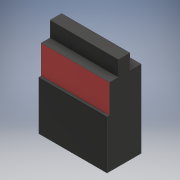
# Autodesk Inventor part: Battery_278Wh
Saved by Autodesk Inventor 2017 (Build 210142000, 142)
## iProperties
Created: 2019-06-03
Part Number: Battery_278Wh
Material: ABS Plastic
Document SubType Name: Modeling
Designer: Dell
Density: 1.06 g/cm^3
Appearance: Smooth - Black
Author: Dell
Autodesk Inventor part; units mm, degrees
ref_plane "YZ Plane" through (0, 0, 0) normal (1, 0, 0) x (0, 1, 0)
ref_plane "XZ Plane" through (0, 0, 0) normal (0, 1, 0) x (-1, 0, 0)
ref_plane "XY Plane" through (0, 0, 0) normal (0, 0, 1) x (1, 0, 0)
sketch "Sketch1" plane through (0, 0, 0) normal (0, 0, 1) x (1, 0, 0)
  line L0 (0, 0) -> (177.8, 0)
  line L1 (177.8, 0) -> (177.8, 88.9)
  line L2 (177.8, 88.9) -> (0, 88.9)
  line L3 (0, 88.9) -> (0, 0)
  dimension "d0" = 88.9
  dimension "d1" = 177.8
  constraints: 8 end point, 2 parallel, 1 horizontal, 1 perpendicular
  measures "d0" distance of L2.end L0.start
  measures "d1" distance of L1.end L2.end
extrude "Extrusion1" add sketch "Sketch1" along normal blind 241.3
sketch "Sketch2" plane through (0, 0, 0) normal (0, -1, 0) x (1, 0, 0)
  line L0 (0, 0) -> (0, 241.3) projected
  line L1 (177.8, 0) -> (177.8, 241.3) projected
  line L2 (0, 203.2) -> (177.8, 203.2)
  line L3 (177.8, 203.2) -> (177.8, 127)
  line L4 (177.8, 127) -> (0, 127)
  line L5 (0, 127) -> (0, 203.2)
  line L6 (0, 0) -> (177.8, 0) projected
  dimension "d4" = 203.2
  dimension "d5" = 127
  constraints: 8 end point, 2 parallel, 2 point on line, 1 horizontal, 1 perpendicular
  measures "d4" distance between parallel lines of L6 L2
  measures "d5" distance between parallel lines of L6 L4
extrude "Extrusion2" cut sketch "Sketch2" against normal blind 6.35 contours L0 L2 L1 L4
sketch "Sketch3" plane through (0, 0, 241.3) normal (0, 0, 1) x (1, 0, 0)
  line L0 (177.8, 0) -> (177.8, 88.9) projected
  line L1 (0, 0) -> (177.8, 0)
  line L2 (177.8, 0) -> (177.8, 29.45)
  line L3 (177.8, 29.45) -> (0, 29.45)
  line L4 (0, 29.45) -> (0, 0)
  line L5 (0, 88.9) -> (0, 0) projected
  line L6 (0, 88.9) -> (177.8, 88.9)
  line L7 (177.8, 88.9) -> (177.8, 59.45)
  line L8 (177.8, 59.45) -> (0, 59.45)
  line L9 (0, 59.45) -> (0, 88.9)
  line L10 (88.9, 29.45) -> (88.9, 59.45) construction
  point P0 (0, 44.45)
  point P1 (88.9, 44.45)
  dimension "d8" = 30
  constraints: 18 end point, 4 midpoint, 4 parallel, 2 horizontal, 2 perpendicular, 2 point on line, 1 horizontal alignment
  measures "d8" distance between parallel lines of L8 L3
extrude "Extrusion3" cut sketch "Sketch3" against normal blind 40 contours L1 L4 L3 L0 | L8 L5 L6 L0
body "Solid1"
